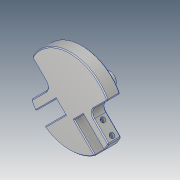
# Autodesk Inventor part: 200-20-ROCKER-CONNECTOR-01
Saved by Autodesk Inventor 2018.1 (Build 221171000, 171)
## iProperties
Created: 2017-10-30
Part Number: 200-20-ROCKER-CONNECTOR-01
Material: Aluminium 6061
Document SubType Name: Modeling
Designer: Martin Fees
Density: 2.7 g/cm^3
Appearance: Aluminium - flach
Author: Martin Fees
Autodesk Inventor part; units mm, degrees
ref_plane "YZ Plane" through (0, 0, 0) normal (1, 0, 0) x (0, 1, 0)
ref_plane "XZ Plane" through (0, 0, 0) normal (0, 1, 0) x (-1, 0, 0)
ref_plane "XY Plane" through (0, 0, 0) normal (0, 0, 1) x (1, 0, 0)
derived "200-10-ROCKER-BEARING-01.ipt"
sketch "Skizze_Lagersitz" plane through (0, 0, 0) normal (1, 0, 0) x (0, 1, 0)
  line L0 (-12.5, 36) -> (32.5, 36)
  line L1 (-12.5, -36) -> (-12.5, 36)
  line L2 (-17.5, 32.25) -> (-12.5, 32.25)
  line L3 (-17.5, -32.25) -> (-17.5, 32.25)
  line L4 (-32.5, 18) -> (-17.5, 18)
  line L5 (-32.5, -18) -> (-17.5, -18)
  line L6 (-17.5, -32.25) -> (-12.5, -32.25)
  line L7 (-12.5, -36) -> (32.5, -36)
  line L8 (32.5, 36) -> (32.5, -36)
  line L9 (32.5, 50) -> (32.5, -50)
  line L10 (30, -50) -> (30, 0)
  line L11 (-32.5, -18) -> (-32.5, 18)
  line L12 (-32.5, 50) -> (-32.5, -50)
  line L13 (-32.5, -50) -> (-32.5, 50)
  line L14 (-12.5, -36) -> (-12.5, 36)
  point P0 (0, 0)
  point P1 (30, 86)
  point P2 (30, 14)
  point P3 (-30, 32)
  point P4 (-30, 68)
sketch "Skizze4" plane through (0, 0, 0) normal (1, 0, 0) x (0, 1, 0)
  line L0 (-93.26, 0) -> (53.46, 0) projected
  line L1 (-12.5, -36) -> (-12.5, 36) construction
  line L2 (-32.5, -18) -> (-32.5, 18) construction
  line L3 (22.7, 0) -> (22.7, 15)
  line L4 (22.7, 15) -> (-12.5, 15)
  line L5 (17.7, 0) -> (17.7, 36) construction
  line L6 (-12.5, 15) -> (-12.5, 19)
  line L7 (-12.5, 19) -> (-42.3, 19)
  line L8 (-42.3, 19) -> (-42.3, 100)
  line L9 (-42.3, 100) -> (-72.3, 100)
  line L10 (-72.3, 100) -> (-72.3, 0)
  line L11 (-72.3, 0) -> (22.7, 0)
  point P0 (0, 0)
  dimension "d3" = 30.2
  dimension "d4" = 5
  dimension "d5" = 30
  dimension "d6" = 38
  dimension "d7" = 65
  dimension "d8" = 200
  dimension "d9" = 30
  constraints: 18 end point, 5 point on line, 3 perpendicular, 3 vertical, 2 horizontal
  measures "d3" distance between parallel lines of L5 L1
  measures "d4" distance between parallel lines of L3 L5
  measures "d5" diameter of L4 L0
  measures "d6" diameter of L7 L0
  measures "d7" distance from line of L7.end L3
  measures "d8" diameter of L9 L0
  measures "d9" distance of L8.end L9.end
revolve "Grundkoerper" add sketch "Skizze4" angle 360 about axis through (0, 0, 0) along (0, 1, 0)
sketch "Skizze6" plane through (0, -72.3, 0) normal (0, -1, 0) x (1, 0, 0)
  line L0 (0, 0) -> (-70.7107, -70.7107) construction
  circle A0 centre (0, 0) radius 100 projected
  circle A1 centre (0, 0) radius 15 projected
  line L1 (0, 140) -> (0, -140) construction
  line L2 (-60.1041, -81.3173) -> (-81.3173, -60.1041)
  line L3 (-81.3173, -60.1041) -> (-31.8198, -10.6066)
  line L4 (-31.8198, -10.6066) -> (-10.6066, -31.8198)
  line L5 (-10.6066, -31.8198) -> (-60.1041, -81.3173)
  line L6 (0, 0) -> (70.7107, -70.7107) construction
  line L7 (60.1041, -81.3173) -> (81.3173, -60.1041)
  line L8 (81.3173, -60.1041) -> (31.8198, -10.6066)
  line L9 (31.8198, -10.6066) -> (10.6066, -31.8198)
  line L10 (10.6066, -31.8198) -> (60.1041, -81.3173)
  line L11 (-45.9619, 3.5355) -> (-95.4594, -45.9619)
  line L12 (-31.8198, -10.6066) -> (-45.9619, 3.5355) construction
  line L13 (-81.3173, -60.1041) -> (-95.4594, -45.9619) construction
  line L14 (-45.9619, 3.5355) -> (-88.6669, 46.2405)
  line L15 (-88.6669, 46.2405) -> (-138.1644, -3.257)
  line L16 (-138.1644, -3.257) -> (-95.4594, -45.9619)
  line L17 (45.9619, 3.5355) -> (95.4594, -45.9619)
  line L18 (45.9619, 3.5355) -> (88.6669, 46.2405)
  line L19 (88.6669, 46.2405) -> (138.1644, -3.257)
  line L20 (138.1644, -3.257) -> (95.4594, -45.9619)
  dimension "d17" = 30
  dimension "d18" = 30
  dimension "d19" = 90
  dimension "d22" = 20
  constraints: 42 end point, 9 symmetric about line, 6 perpendicular, 3 parallel, 2 point on circle, 1 midpoint, 1 tangent
  measures "d17" distance of L2.end L2.start
  measures "d18" distance from line of A1.centre L4
  measures "d19" angle of L6 L0
  measures "d22" distance between parallel lines of L3 L11
extrude "Ausschnitt_Bosch_30x30" cut sketch "Skizze6" against normal through all contours A0 L17 L18 | A0 L19 L20 L17 | L14 L11 A0 | A0 L11 L16 L15 | L8 L7 A0 | A0 L10 L9 L8 | L7 L10 A0 | L3 L4 L5 A0 | A0 L2 L3 | A0 L5 L2
sketch "Skizze7" plane through (-90.9869, -72.3, -41.4895) normal (-0.7071068, 0, 0.7071068) x (0.7071068, 0, 0.7071068)
  line L0 (63.675, 30) -> (63.675, 0) construction
  line L1 (0, 0) -> (0, 30) construction
  line L2 (63.675, 0) -> (0, 0) construction
  line L3 (0, 30) -> (63.675, 30) construction
  line L4 (0, 15) -> (63.675, 15) construction
  line L5 (63.675, 30) -> (-5.1936, 30) projected
  point P0 (93.675, 72.3)
  point P1 (40, 15)
  point P2 (10, 15)
  dimension "d27" = 30
  dimension "d35" = 10
  constraints: 2 end point, 2 midpoint, 2 point on line
  measures "d27" distance of point (10, 15) point (40, 15)
  measures "d35" distance from line of L1 point (10, 15)
hole "BOH_M6_ISO4762" at (-62.7027, -57.3, -13.2052) at (-83.9159, -57.3, -34.4184) direction (0.7071068, 0, -0.7071068) diameter 6.6 end up to face face through (-64.2848, -52.3, -43.0716) facing (0.7071068, 0, -0.7071068) counterbore diameter 11 counterbore depth 6.4
mirror "Spiegeln1" about plane through (0, 0, 0) normal (1, 0, 0) of "BOH_M6_ISO4762"
sketch "Skizze8" plane through (0, 22.7, 0) normal (0, 1, 0) x (1, 0, 0)
  circle A0 centre (0, 0) radius 15 construction
  constraints: 1 coincident
hole "BOH_M6x1" at (0, 22.7, 0) direction (0, -1, 0) diameter 4.917 depth 19.1 tip angle 118 countersink diameter 6 countersink angle 90 thread size "M6x1" class "6H" standard "ISO Metric profile"
fillet "Rundung1" radius 15 2 edges at (-45.9619, -57.3, 3.5355) (45.9619, -57.3, 3.5355)
chamfer "Fase_Allgemein" distance 2 angle 45 40 edges at (-90.9869, -57.3, -41.4895) (-80.5173, -57.3, -59.3041) (-59.3041, -57.3, -80.5173) (59.3041, -57.3, -80.5173) (80.5173, -57.3, -59.3041) (90.9869, -57.3, -41.4895) (88.6669, -57.3, 46.2405) (-88.6669, -57.3, 46.2405) (-56.1685, -72.3, -34.9553) (-21.2132, -72.3, -21.2132) (-34.9553, -72.3, -56.1685) (-34.9553, -42.3, -56.1685) (-21.2132, -42.3, -21.2132) (-56.1685, -42.3, -34.9553) (34.9553, -72.3, -56.1685) (21.2132, -72.3, -21.2132) (56.1685, -72.3, -34.9553) (34.9553, -42.3, -56.1685) (21.2132, -42.3, -21.2132) (56.1685, -42.3, -34.9553) (0, -72.3, -100) (0, -42.3, -100) (-86.2135, -72.3, -50.6679) (-86.2135, -42.3, -50.6679) (86.2135, -72.3, -50.6679) (86.2135, -42.3, -50.6679) (72.6177, -72.3, 30.1913) (52.1751, -72.3, 3.5355) (73.7777, -72.3, -24.2803) (0, -72.3, 100) (-52.1751, -72.3, 3.5355) (-72.6177, -72.3, 30.1913) (-73.7777, -72.3, -24.2803) (73.7777, -42.3, -24.2803) (52.1751, -42.3, 3.5355) (72.6177, -42.3, 30.1913) (0, -42.3, 100) (-72.6177, -42.3, 30.1913) (-52.1751, -42.3, 3.5355) (-73.7777, -42.3, -24.2803)
chamfer "Fase_Achse" distance 0.5 angle 45 2 edges at (0, 22.7, -15) (0, -12.5, -19)
chamfer "Fase_Achse_2" distance 2 angle 45 1 edges at (0, -42.3, -19)
sketch "Skizze10" plane through (0, 22.7, 0) normal (0, 1, 0) x (1, 0, 0)
  point P0 (0, 0)
